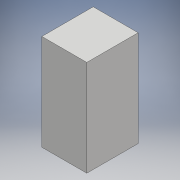
# Autodesk Inventor part: F-nose
Saved by Autodesk Inventor 2018.1 (Build 221171000, 171)
## iProperties
Created: 2017-11-03
Part Number: F-nose
Material: 一般
Document SubType Name: Modeling
Designer: ku_sk
Density: 1 g/cm^3
Appearance: 既定
Author: ku_sk
Autodesk Inventor part; units mm, degrees
ref_plane "YZ Plane" through (0, 0, 0) normal (1, 0, 0) x (0, 1, 0)
ref_plane "XZ Plane" through (0, 0, 0) normal (0, 1, 0) x (-1, 0, 0)
ref_plane "XY Plane" through (0, 0, 0) normal (0, 0, 1) x (1, 0, 0)
sketch "スケッチ1" plane through (0, 0, 0) normal (0, 0, 1) x (1, 0, 0)
  line L0 (-265, 303) -> (265, 303)
  line L1 (265, 303) -> (265, -303)
  line L2 (265, -303) -> (-265, -303)
  line L3 (-265, -303) -> (-265, 303)
  line L4 (0, -424.2) -> (0, 424.2) projected
  line L5 (-371, 0) -> (371, 0) projected
  point P0 (0, 0)
  point P1 (0, 303)
  point P2 (-265, 0)
  dimension "d2" = 530
  dimension "d3" = 606
  constraints: 8 end point, 2 midpoint, 2 parallel, 2 point on line, 1 horizontal, 1 perpendicular
  measures "d2" distance of L0.start L0.end
  measures "d3" distance of L2.end L0.start
extrude "押し出し1" add sketch "スケッチ1" along normal mid plane 1132
